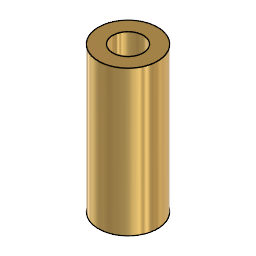
Koi Mp3 Full Assembly (Autodesk Fusion 360 archive; units mm, degrees)
design "brass 10mm standoffs"
part number: 2026-06-01-13-56-33-233
Autodesk Fusion 360 part; units mm, degrees
sketch "Sketch1" plane through (0, 0, 0) normal (0, 0, 1) x (1, 0, 0)
  circle A0 centre (0, 0) radius 1.05
  circle A1 centre (0, 0) radius 2.032
  dimension "d1" = 2.1
  constraint coincident A0.centre A1.centre
  measures "d1" diameter of A0
extrude "Extrude1" add sketch "Sketch1" along normal blind 10

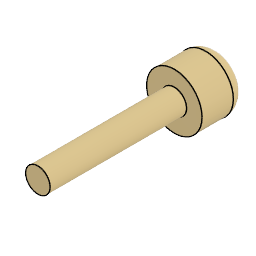
design "rubber button"
part number: 2026-06-01-19-31-11-983
Autodesk Fusion 360 part; units mm, degrees
sketch "Sketch2" plane through (0, 0, 0) normal (0, -1, 0) x (1, 0, 0)
  circle A0 centre (0, 0) radius 0.9974
  circle A1 centre (0, 0) radius 2.2479
  constraint coincident A0.centre A1.centre
extrude "Extrude1" add sketch "Sketch2" along normal blind 7.25 contours A0
extrude "Extrude2" add 1 faces at (-0.2437, -7.25, 0.2261) along direction (0, -1, 0) blind 7.366
extrude "Extrude4" cut 1 faces at (-0.2437, -14.616, 0.2261) along direction (0, 1, 0) blind 2.54
sketch "Sketch3" plane through (0, 0, 0) normal (0, 1, 0) x (-1, 0, 0)
  circle A0 centre (0, 0) radius 0.9974
  circle A1 centre (0, 0) radius 2.2479
  dimension "d14" = 4.4958
  constraint concentric A0 A1
  measures "d14" diameter of A1
extrude "Extrude5" add sketch "Sketch3" along normal blind 3.81 contours A0 | A1
extrude "Extrude6" add 1 faces at (-1.819, 0, -0.1612) along direction (0, -1, 0) blind 1.016
extrude "Extrude7" cut 1 faces at (-0.7569, 3.81, -0.3251) along direction (0, -1, 0) blind 1.27
fillet "Fillet1" radius 1.016 1 edges at (2.0958, 2.54, 0.8129)
